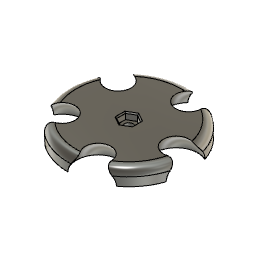
domekit_gheleguen_hub_x5_up_v2 (Autodesk Fusion 360 design; units mm, degrees)
Autodesk Fusion 360 part; units mm, degrees
sketch "Esquisse1" plane through (0, 0, 1) normal (0, 0, 1) x (1, 0, 0)
  circle A0 centre (0, 0) radius 27.75
  dimension "d1" = 55.5
  constraint coincident A0.centre origin
  measures "d1" diameter of A0
extrude "Extrusion1" add sketch "Esquisse1" along normal blind 7.5
ref_plane "Plan de construction3" through (0, 0, 0.5) normal (0, 0, -1) x (-1, 0, 0)
sketch "Esquisse2" plane through (0, 0, 0.5) normal (0, 0, -1) x (1, 0, 0)
  circle A0 centre (22, 0) radius 9.995
  circle A1 centre (0, 0) radius 27.75
  circle A2 centre (0, 0) radius 27.75
  dimension "d4" = 19.99
  dimension "d8" = 22
  measures "d4" diameter of A0
  measures "d8" distance of A1.centre A0.centre
sphere "SpherePrimitive1" cut diameter 19.9 placed x (1, 0, 0) y (0, -1, 0) z (0, 0, -1) at (22, 0, 0.5)
pattern_circular "Réseau C1" count 5 over 360 about axis through (0, 0, 1.75) along (0, 0, 1) of "SpherePrimitive1"
fillet "Congé1" chord length 5 10 edges at (22.4502, -16.311, 8.5) (22.4502, 16.311, 8.5) (-8.5752, 26.3918, 8.5) (-27.75, 0, 8.5) (-8.5752, -26.3918, 8.5) (-8.5752, -26.3918, 8.5) (22.4502, -16.311, 8.5) (22.4502, 16.311, 8.5) (-8.5752, 26.3918, 8.5) (-27.75, 0, 8.5)
hole "Perçage1" at (0, 0, 0.5) direction (0, 0, 1) diameter 4.3 depth 13 tip angle 180
sketch "Esquisse4" plane through (0, 0, 8.5) normal (0, 0, 1) x (-1, 0, 0)
  circle A0 centre (0, 0) radius 2.15
  spline S0 degree 3 poles (-1.8361, 24.1448) (-0.9987, 24.2084) (-0.1568, 24.2285) (2.9886, 24.1398) (5.2871, 23.7427) (7.4827, 23.0293) (9.6782, 22.3159) (11.7712, 21.2862) (14.368, 19.5091) (15.0373, 18.998) (15.6774, 18.4543) knots -2.328527 -2.328527 -2.328527 -2.328527 -2.076596 -2.076596 -1.384397 -1.384397 -1.384397 -0.692199 -0.692199 -0.440268 -0.440268 -0.440268 -0.440268
  arc A1 (-12.7065, 20.6127) -> (-1.8361, 24.1448) centre (-6.7984, 20.9232) ccw
  spline S1 degree 3 poles (-23.5304, 5.7149) (-23.3322, 6.531) (-23.0911, 7.3379) (-22.0348, 10.302) (-20.9468, 12.3652) (-19.5899, 14.2329) (-18.233, 16.1006) (-16.6069, 17.7728) (-14.1143, 19.6935) (-13.4214, 20.172) (-12.7065, 20.6127) knots -2.328527 -2.328527 -2.328527 -2.328527 -2.076596 -2.076596 -1.384397 -1.384397 -1.384397 -0.692199 -0.692199 -0.440268 -0.440268 -0.440268 -0.440268
  arc A2 (-23.5304, -5.7149) -> (-23.5304, 5.7149) centre (-22, 0) ccw
  spline S2 degree 3 poles (-12.7065, -20.6127) (-13.4214, -20.172) (-14.1143, -19.6935) (-16.6069, -17.7728) (-18.233, -16.1006) (-19.5899, -14.2329) (-20.9468, -12.3652) (-22.0348, -10.302) (-23.0911, -7.3379) (-23.3322, -6.531) (-23.5304, -5.7149) knots -2.328527 -2.328527 -2.328527 -2.328527 -2.076596 -2.076596 -1.384397 -1.384397 -1.384397 -0.692199 -0.692199 -0.440268 -0.440268 -0.440268 -0.440268
  arc A3 (-1.8361, -24.1448) -> (-12.7065, -20.6127) centre (-6.7984, -20.9232) ccw
  spline S3 degree 3 poles (15.6774, -18.4543) (15.0373, -18.998) (14.368, -19.5091) (11.7712, -21.2862) (9.6782, -22.3159) (7.4827, -23.0293) (5.2871, -23.7427) (2.9886, -24.1398) (-0.1568, -24.2285) (-0.9987, -24.2084) (-1.8361, -24.1448) knots -2.328527 -2.328527 -2.328527 -2.328527 -2.076596 -2.076596 -1.384397 -1.384397 -1.384397 -0.692199 -0.692199 -0.440268 -0.440268 -0.440268 -0.440268
  arc A4 (22.3956, -9.2074) -> (15.6774, -18.4543) centre (17.7984, -12.9313) ccw
  spline S4 degree 3 poles (22.3956, 9.2074) (22.715, 8.4306) (22.9942, 7.6362) (23.8819, 4.6173) (24.2145, 2.3086) (24.2145, 0) (24.2145, -2.3086) (23.8819, -4.6173) (22.9942, -7.6362) (22.715, -8.4306) (22.3956, -9.2074) knots -2.328527 -2.328527 -2.328527 -2.328527 -2.076596 -2.076596 -1.384397 -1.384397 -1.384397 -0.692199 -0.692199 -0.440268 -0.440268 -0.440268 -0.440268
  arc A5 (15.6774, 18.4543) -> (22.3956, 9.2074) centre (17.7984, 12.9313) ccw
  line L0 (-3.5, -2.0207) -> (0, -4.0415)
  line L1 (0, -4.0415) -> (3.5, -2.0207)
  line L2 (3.5, -2.0207) -> (3.5, 2.0207)
  line L3 (3.5, 2.0207) -> (0, 4.0415)
  line L4 (0, 4.0415) -> (-3.5, 2.0207)
  line L5 (-3.5, 2.0207) -> (-3.5, -2.0207)
  dimension "d24" = 3.5
  constraint coincident A0.centre origin
  measures "d24" distance of A0.centre L5
extrude "Extrusion2" cut sketch "Esquisse4" against normal blind 3 contours L0 L1 L2 L3 L4 L5
chamfer "Chanfrein1" distance 0.5 angle 45 6 edges at (-1.75, 3.0311, 8.5) (1.75, 3.0311, 8.5) (3.5, 0, 8.5) (1.75, -3.0311, 8.5) (-1.75, -3.0311, 8.5) (-3.5, 0, 8.5)
